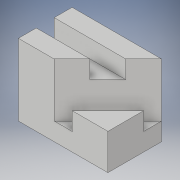
# Autodesk Inventor part: 零件17
Saved by Autodesk Inventor 2019 (Build 230136000, 136)
## iProperties
Created: 2020-09-18
Part Number: 零件17
Material: 一般
Document SubType Name: Modeling
Designer: jay
Density: 1 g/cm^3
Appearance: 預設
Author: jay
Autodesk Inventor part; units mm, degrees
ref_plane "YZ Plane" through (0, 0, 0) normal (1, 0, 0) x (0, 1, 0)
ref_plane "XZ Plane" through (0, 0, 0) normal (0, 1, 0) x (-1, 0, 0)
ref_plane "XY Plane" through (0, 0, 0) normal (0, 0, 1) x (1, 0, 0)
sketch "草圖1" plane through (0, 0, 0) normal (0, 0, 1) x (1, 0, 0)
  line L0 (0, 0) -> (50, 0)
  line L1 (50, 0) -> (50, 40)
  line L2 (50, 40) -> (0, 40)
  line L3 (0, 40) -> (0, 0)
  dimension "d0" = 50
  dimension "d1" = 40
  constraints: 8 end point, 2 parallel, 1 horizontal, 1 perpendicular
  measures "d0" distance of L1.end L2.end
  measures "d1" distance of L2.end L0.start
extrude "擠出1" add sketch "草圖1" along normal blind 30
sketch "草圖2" plane through (0, 40, 0) normal (0, 1, 0) x (1, 0, 0)
  line L0 (50, 0) -> (50, -30) projected
  line L1 (0, -20) -> (50, -20)
  line L2 (50, -20) -> (50, -10)
  line L3 (50, -10) -> (0, -10)
  line L4 (0, -10) -> (0, -20)
  line L5 (50, 0) -> (0, 0) projected
  line L6 (0, 0) -> (0, -30) projected
  dimension "d4" = 10
  dimension "d5" = 10
  constraints: 8 end point, 2 parallel, 1 collinear, 1 horizontal, 1 perpendicular, 1 point on line
  measures "d4" distance between parallel lines of L5 L3
  measures "d5" distance of L3.end L1.start
extrude "擠出2" cut sketch "草圖2" against normal blind 10 contours L0 L1 L4 L3
sketch "草圖3" plane through (0, 40, 30) normal (0, 1, 0) x (1, 0, 0)
  line L0 (20, 0) -> (50, 30)
  line L1 (50, 30) -> (50, 20) projected
  line L2 (50, 30) -> (50, 0)
  line L3 (50, 0) -> (20, 0)
  line L4 (50, 30) -> (0, 30) projected
  line L5 (50, 10) -> (50, 0) projected
  line L6 (50, 0) -> (0, 0) projected
  line L7 (30, 0) -> (50, 20)
  dimension "d8" = 30
  dimension "d9" = 10
  dimension "d10" = 10
  constraints: 8 end point, 2 point on line, 1 collinear, 1 perpendicular, 1 vertical
  measures "d8" distance from line of L2 L0.start
  measures "d9" distance of L0.end L7.end
  measures "d10" distance of L0.start L7.start
extrude "擠出3" cut sketch "草圖3" against normal blind 30 contours L0 L1 L7 L3
sketch "草圖4" plane through (50, 40, 30) normal (0, 1, 0) x (1, 0, 0)
  line L0 (-10, 10) -> (-20, 0) projected
  line L1 (0, 0) -> (-20, 0) projected
  line L2 (0, 10) -> (0, 0) projected
  line L3 (0, 10) -> (-10, 10) projected
  line L4 (0, 20) -> (-10, 10) projected
  line L5 (0, 10) -> (-10, 10) projected
  line L6 (0, 20) -> (0, 10) projected
  point P0 (-50, 30)
extrude "擠出4" cut sketch "草圖4" against normal blind 20
